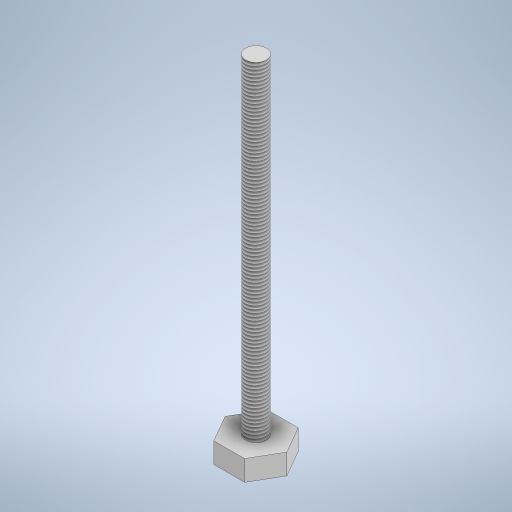
# Autodesk Inventor part: Bolt
Saved by Autodesk Inventor 2024 (Build 280153020, 153B)
## iProperties
Created: 2023-08-30
Part Number: Bolt
Material: Generic
Document SubType Name: Modeling
Designer: Victoria
Density: 1 g/cm^3
Appearance: Default
Author: Victoria
Autodesk Inventor part; units mm, degrees
ref_plane "YZ Plane" through (0, 0, 0) normal (1, 0, 0) x (0, 1, 0)
ref_plane "XZ Plane" through (0, 0, 0) normal (0, 1, 0) x (-1, 0, 0)
ref_plane "XY Plane" through (0, 0, 0) normal (0, 0, 1) x (1, 0, 0)
sketch "Sketch1" plane through (0, 0, 0) normal (0, 1, 0) x (-1, 0, 0)
  circle A0 centre (0, 0) radius 7.5
  dimension "d0" = 15
  constraints: 1 centre point, 1 coincident
  measures "d0" diameter of A0
extrude "Extrusion1" add sketch "Sketch1" along normal blind 5
sketch "Sketch2" plane through (0, 5, 0) normal (0, 1, 0) x (1, 0, 0)
  circle A0 centre (0, 0) radius 2.5
  dimension "d3" = 5
  constraints: 1 centre point, 1 coincident
  measures "d3" diameter of A0
extrude "Extrusion2" add sketch "Sketch2" along normal blind 80
thread "Thread1" size "M5x0.8" class "6g" standard "ANSI Metric M Profile" length 80
sketch "Sketch3" plane through (0, 0, 0) normal (0, -1, 0) x (1, 0, 0)
  circle A0 centre (0, 0) radius 7.5 projected
  line L0 (-7.5, 0) -> (0, 0)
  line L1 (0, 0) -> (-3.75, -6.4952)
  line L2 (0, 0) -> (3.75, -6.4952)
  line L3 (0, 0) -> (7.5, 0) construction
  line L4 (0, 0) -> (3.75, 6.4952)
  line L5 (0, 0) -> (7.5, 0) construction
  line L6 (0, 0) -> (-3.75, 6.4952)
  line L7 (0, 0) -> (7.5, 0) construction
  line L8 (-7.5, 0) -> (-3.75, -6.4952)
  line L9 (-3.75, -6.4952) -> (3.75, -6.4952)
  line L10 (3.75, -6.4952) -> (7.5, 0)
  line L11 (7.5, 0) -> (3.75, 6.4952)
  line L12 (3.75, 6.4952) -> (-3.75, 6.4952)
  line L13 (-3.75, 6.4952) -> (-7.5, 0)
  point P0 (7.5, 0)
  point P1 (7.5, 0)
  dimension "d8" = 60
  dimension "d9" = 60
  dimension "d10" = 60
  dimension "d11" = 120
  constraints: 28 end point, 5 point on circle, 4 horizontal, 3 equal length, 1 parallel
  measures "d8" angle of L0 L1
  measures "d9" angle of L2 L3
  measures "d10" angle of L5 L4
  measures "d11" angle of L7 L6
extrude "Extrusion3" cut sketch "Sketch3" against normal through all contours L11 A0 | A0 L10 | L12 A0 | A0 L9 | L13 A0 | A0 L8
body "Solid1"
